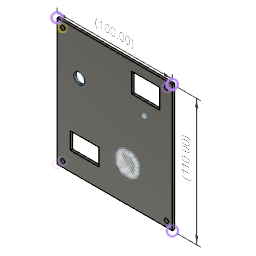
enclosure (Autodesk Fusion 360 archive; units mm, degrees)
design "Untitled"
part number: 2025-12-20-12-13-13-298
Autodesk Fusion 360 part; units mm, degrees
sketch "Sketch1" plane through (0, 0, 0) normal (0, 1, 0) x (1, 0, 0)
  line L0 (-50, -50) -> (40, -50)
  line L1 (40, -50) -> (40, 50)
  line L2 (40, 50) -> (-50, 50)
  line L3 (-50, 50) -> (-50, -50)
  dimension "d1" = 90
  dimension "d2" = 100
  constraint horizontal L0
  constraint vertical L1
  constraint horizontal L2
  constraint vertical L3
  measures "d1" distance of L0.start L0.end
  measures "d2" distance of L0.start L2.end
sketch "Sketch2" plane through (0, 0, 0) normal (0, 1, 0) x (1, 0, 0)
sketch "Sketch3" plane through (0, 0, 0) normal (0, 1, 0) x (1, 0, 0)
sketch "Sketch4" plane through (0, 0, 0) normal (0, 1, 0) x (1, 0, 0)
  line L0 (-43.399, 24.1645) -> (-18.699, 24.1645)
  line L1 (-18.699, 24.1645) -> (-18.699, 38.7645)
  line L2 (-18.699, 38.7645) -> (-43.399, 38.7645)
  line L3 (-43.399, 38.7645) -> (-43.399, 24.1645)
  dimension "d10" = 24.7
  dimension "d11" = 14.6
  constraint horizontal L0
  constraint vertical L1
  constraint horizontal L2
  constraint vertical L3
  measures "d10" distance of L0.start L0.end
  measures "d11" distance of L0.start L2.end
sketch "Sketch5" plane through (0, 0, 0) normal (0, 1, 0) x (1, 0, 0)
  circle A0 centre (-35.7, -19.12) radius 4.784
  circle A1 centre (0, 17) radius 0.35
  circle A2 centre (1, 18) radius 0.35
  circle A3 centre (2, 19) radius 0.35
  circle A4 centre (3, 20) radius 0.35
  circle A5 centre (4, 21) radius 0.35
  circle A6 centre (5, 22) radius 0.35
  circle A7 centre (6, 23) radius 0.35
  circle A8 centre (7, 24) radius 0.35
  circle A9 centre (8, 25) radius 0.35
  circle A10 centre (9, 26) radius 0.35
  circle A11 centre (10, 27) radius 0.35
  circle A12 centre (11, 28) radius 0.35
  circle A13 centre (12, 29) radius 0.35
  circle A14 centre (13, 30) radius 0.35
  circle A15 centre (1.9315, 15.9772) radius 0.35
  circle A16 centre (2.9315, 16.9772) radius 0.35
  circle A17 centre (3.9315, 17.9772) radius 0.35
  circle A18 centre (4.9315, 18.9772) radius 0.35
  circle A19 centre (5.9315, 19.9772) radius 0.35
  circle A20 centre (6.9315, 20.9772) radius 0.35
  circle A21 centre (7.9315, 21.9772) radius 0.35
  circle A22 centre (8.9315, 22.9772) radius 0.35
  circle A23 centre (1, 18) radius 0.35
  circle A24 centre (11.9315, 25.9772) radius 0.35
  circle A25 centre (10.9315, 24.9772) radius 0.35
  circle A26 centre (9.9315, 23.9772) radius 0.35
  circle A27 centre (12.9315, 26.9772) radius 0.35
  circle A28 centre (13.9315, 27.9772) radius 0.35
  circle A29 centre (13.9315, 24.9772) radius 0.35
  circle A30 centre (12.9315, 23.9772) radius 0.35
  circle A31 centre (11.9315, 22.9772) radius 0.35
  circle A32 centre (10.9315, 21.9772) radius 0.35
  circle A33 centre (9.9315, 20.9772) radius 0.35
  circle A34 centre (8.9315, 19.9772) radius 0.35
  circle A35 centre (7.9315, 18.9772) radius 0.35
  circle A36 centre (6.9315, 17.9772) radius 0.35
  circle A37 centre (5.9315, 16.9772) radius 0.35
  circle A38 centre (4.9315, 15.9772) radius 0.35
  circle A39 centre (3.9315, 14.9772) radius 0.35
  circle A40 centre (14.9315, 25.9772) radius 0.35
  circle A41 centre (6.9315, 14.9772) radius 0.35
  circle A42 centre (7.9315, 15.9772) radius 0.35
  circle A43 centre (8.9315, 16.9772) radius 0.35
  circle A44 centre (9.9315, 17.9772) radius 0.35
  circle A45 centre (10.9315, 18.9772) radius 0.35
  circle A46 centre (11.9315, 19.9772) radius 0.35
  circle A47 centre (12.9315, 20.9772) radius 0.35
  circle A48 centre (13.9315, 21.9772) radius 0.35
  circle A49 centre (14.9315, 22.9772) radius 0.35
  circle A50 centre (14.9315, 19.9772) radius 0.35
  circle A51 centre (13.9315, 18.9772) radius 0.35
  circle A52 centre (12.9315, 17.9772) radius 0.35
  circle A53 centre (11.9315, 16.9772) radius 0.35
  circle A54 centre (10.9315, 15.9772) radius 0.35
  circle A55 centre (9.9315, 14.9772) radius 0.35
  circle A56 centre (10.9315, 30.9772) radius 0.35
  circle A57 centre (9.9315, 29.9772) radius 0.35
  circle A58 centre (8.9315, 28.9772) radius 0.35
  circle A59 centre (7.9315, 27.9772) radius 0.35
  circle A60 centre (6.9315, 26.9772) radius 0.35
  circle A61 centre (5.9315, 25.9772) radius 0.35
  circle A62 centre (4.9315, 24.9772) radius 0.35
  circle A63 centre (3.9315, 23.9772) radius 0.35
  circle A64 centre (2.9315, 22.9772) radius 0.35
  circle A65 centre (1.9315, 21.9772) radius 0.35
  circle A66 centre (0.9315, 20.9772) radius 0.35
  circle A67 centre (-0.0685, 19.9772) radius 0.35
  circle A68 centre (-1.0685, 18.9772) radius 0.35
  circle A69 centre (-2.0685, 20.9772) radius 0.35
  circle A70 centre (-1.0685, 21.9772) radius 0.35
  circle A71 centre (-0.0685, 22.9772) radius 0.35
  circle A72 centre (0.9315, 23.9772) radius 0.35
  circle A73 centre (1.9315, 24.9772) radius 0.35
  circle A74 centre (2.9315, 25.9772) radius 0.35
  circle A75 centre (3.9315, 26.9772) radius 0.35
  circle A76 centre (4.9315, 27.9772) radius 0.35
  circle A77 centre (5.9315, 28.9772) radius 0.35
  circle A78 centre (6.9315, 29.9772) radius 0.35
  circle A79 centre (7.9315, 30.9772) radius 0.35
  circle A80 centre (8.9315, 31.9772) radius 0.35
  circle A81 centre (-2.0685, 23.9772) radius 0.35
  circle A82 centre (-1.0685, 24.9772) radius 0.35
  circle A83 centre (-0.0685, 25.9772) radius 0.35
  circle A84 centre (0.9315, 26.9772) radius 0.35
  circle A85 centre (1.9315, 27.9772) radius 0.35
  circle A86 centre (2.9315, 28.9772) radius 0.35
  circle A87 centre (3.9315, 29.9772) radius 0.35
  circle A88 centre (4.9315, 30.9772) radius 0.35
  circle A89 centre (5.9315, 31.9772) radius 0.35
  circle A90 centre (-2.0685, 26.9772) radius 0.35
  circle A91 centre (-1.0685, 27.9772) radius 0.35
  circle A92 centre (-0.0685, 28.9772) radius 0.35
  circle A93 centre (0.9315, 29.9772) radius 0.35
  circle A94 centre (1.9315, 30.9772) radius 0.35
  circle A95 centre (2.9315, 31.9772) radius 0.35
  dimension "d16" = 9.568
  dimension "d20" = 0.7
  dimension "d21" = 0.7
  dimension "d22" = 0.7
  dimension "d23" = 0.7
  dimension "d24" = 0.7
  dimension "d25" = 0.7
  dimension "d26" = 0.7
  dimension "d27" = 0.7
  dimension "d28" = 0.7
  dimension "d29" = 0.7
  dimension "d30" = 0.7
  dimension "d31" = 0.7
  dimension "d32" = 0.7
  dimension "d33" = 0.7
  dimension "d34" = 0.7
  dimension "d35" = 0.7
  dimension "d36" = 0.7
  dimension "d37" = 0.7
  dimension "d38" = 0.7
  dimension "d39" = 0.7
  dimension "d40" = 0.7
  dimension "d41" = 0.7
  dimension "d42" = 0.7
  dimension "d43" = 0.7
  dimension "d44" = 0.7
  dimension "d45" = 0.7
  dimension "d46" = 0.7
  dimension "d47" = 0.7
  dimension "d48" = 0.7
  dimension "d49" = 0.7
  dimension "d50" = 0.7
  dimension "d51" = 0.7
  dimension "d52" = 0.7
  dimension "d53" = 0.7
  dimension "d54" = 0.7
  dimension "d55" = 0.7
  dimension "d56" = 0.7
  dimension "d57" = 0.7
  dimension "d58" = 0.7
  dimension "d59" = 0.7
  dimension "d60" = 0.7
  dimension "d61" = 0.7
  dimension "d62" = 0.7
  dimension "d63" = 0.7
  dimension "d64" = 0.7
  dimension "d65" = 0.7
  dimension "d66" = 0.7
  dimension "d67" = 0.7
  dimension "d68" = 0.7
  dimension "d71" = 0.7
  dimension "d72" = 0.7
  dimension "d73" = 0.7
  dimension "d74" = 0.7
  dimension "d75" = 0.7
  dimension "d76" = 0.7
  dimension "d77" = 0.7
  dimension "d78" = 0.7
  dimension "d79" = 0.7
  dimension "d80" = 0.7
  dimension "d81" = 0.7
  dimension "d82" = 0.7
  dimension "d83" = 0.7
  dimension "d84" = 0.7
  dimension "d85" = 0.7
  dimension "d86" = 0.7
  dimension "d87" = 0.7
  dimension "d88" = 0.7
  dimension "d89" = 0.7
  dimension "d90" = 0.7
  dimension "d91" = 0.7
  dimension "d92" = 0.7
  dimension "d93" = 0.7
  dimension "d94" = 0.7
  dimension "d95" = 0.7
  dimension "d96" = 0.7
  dimension "d97" = 0.7
  dimension "d98" = 0.7
  dimension "d99" = 0.7
  dimension "d100" = 0.7
  dimension "d101" = 0.7
  dimension "d102" = 0.7
  dimension "d103" = 0.7
  dimension "d104" = 0.7
  dimension "d105" = 0.7
  dimension "d106" = 0.7
  dimension "d107" = 0.7
  dimension "d108" = 0.7
  dimension "d109" = 0.7
  dimension "d110" = 0.7
  dimension "d111" = 0.7
  dimension "d112" = 0.7
  dimension "d113" = 0.7
  dimension "d114" = 0.7
  dimension "d115" = 0.7
  dimension "d116" = 0.7
  measures "d16" diameter of A0
  measures "d20" diameter of A1
  measures "d21" diameter of A2
  measures "d22" diameter of A3
  measures "d23" diameter of A4
  measures "d24" diameter of A5
  measures "d25" diameter of A6
  measures "d26" diameter of A7
  measures "d27" diameter of A8
  measures "d28" diameter of A9
  measures "d29" diameter of A10
  measures "d30" diameter of A11
  measures "d31" diameter of A12
  measures "d32" diameter of A13
  measures "d33" diameter of A14
  measures "d34" diameter of A15
  measures "d35" diameter of A16
  measures "d36" diameter of A17
  measures "d37" diameter of A18
  measures "d38" diameter of A19
  measures "d39" diameter of A20
  measures "d40" diameter of A21
  measures "d41" diameter of A22
  measures "d42" diameter of A23
  measures "d43" diameter of A26
  measures "d44" diameter of A25
  measures "d45" diameter of A24
  measures "d46" diameter of A27
  measures "d47" diameter of A28
  measures "d48" diameter of A39
  measures "d49" diameter of A38
  measures "d50" diameter of A37
  measures "d51" diameter of A36
  measures "d52" diameter of A35
  measures "d53" diameter of A34
  measures "d54" diameter of A33
  measures "d55" diameter of A32
  measures "d56" diameter of A31
  measures "d57" diameter of A30
  measures "d58" diameter of A29
  measures "d59" diameter of A40
  measures "d60" diameter of A41
  measures "d61" diameter of A42
  measures "d62" diameter of A43
  measures "d63" diameter of A44
  measures "d64" diameter of A45
  measures "d65" diameter of A46
  measures "d66" diameter of A47
  measures "d67" diameter of A48
  measures "d68" diameter of A49
  measures "d71" diameter of A54
  measures "d72" diameter of A53
  measures "d73" diameter of A52
  measures "d74" diameter of A51
  measures "d75" diameter of A50
  measures "d76" diameter of A55
  measures "d77" diameter of A68
  measures "d78" diameter of A67
  measures "d79" diameter of A66
  measures "d80" diameter of A65
  measures "d81" diameter of A64
  measures "d82" diameter of A63
  measures "d83" diameter of A62
  measures "d84" diameter of A61
  measures "d85" diameter of A60
  measures "d86" diameter of A59
  measures "d87" diameter of A58
  measures "d88" diameter of A57
  measures "d89" diameter of A56
  measures "d90" diameter of A69
  measures "d91" diameter of A70
  measures "d92" diameter of A71
  measures "d93" diameter of A72
  measures "d94" diameter of A73
  measures "d95" diameter of A74
  measures "d96" diameter of A75
  measures "d97" diameter of A76
  measures "d98" diameter of A77
  measures "d99" diameter of A78
  measures "d100" diameter of A79
  measures "d101" diameter of A80
  measures "d102" diameter of A81
  measures "d103" diameter of A82
  measures "d104" diameter of A83
  measures "d105" diameter of A84
  measures "d106" diameter of A85
  measures "d107" diameter of A86
  measures "d108" diameter of A87
  measures "d109" diameter of A88
  measures "d110" diameter of A89
  measures "d111" diameter of A91
  measures "d112" diameter of A92
  measures "d113" diameter of A93
  measures "d114" diameter of A94
  measures "d115" diameter of A95
  measures "d116" diameter of A90
sketch "Sketch6" plane through (0, 0, 0) normal (0, 1, 0) x (1, 0, 0)
  circle A0 centre (20.89, -19.3) radius 0.8835
  dimension "d119" = 1.767
  measures "d119" diameter of A0
sketch "Sketch7" plane through (0, 0, 0) normal (0, 1, 0) x (1, 0, 0)
  line L0 (9.8, -47.2127) -> (34, -47.2127)
  line L1 (34, -47.2127) -> (34, -30.2127)
  line L2 (34, -30.2127) -> (9.8, -30.2127)
  line L3 (9.8, -30.2127) -> (9.8, -47.2127)
  constraint horizontal L0
  constraint vertical L1
  constraint horizontal L2
  constraint vertical L3
extrude "Extrude1" add sketch "Sketch1" along normal blind 2
sketch "Sketch8" plane through (0, 0, 0) normal (0, 1, 0) x (1, 0, 0)
  point P0 (-50, -50)
  point P1 (-50, 50)
  point P2 (40, -50)
  dimension "d131" = 100
  dimension "d132" = 90
  measures "d131" distance of P0 P1
  measures "d132" distance of P0 P2
sketch "Sketch9" plane through (0, 0, 0) normal (0, 1, 0) x (1, 0, 0)
sketch "Sketch10" plane through (0, 0, 0) normal (0, 1, 0) x (1, 0, 0)
sketch "Sketch11" plane through (0, 0, 0) normal (0, 1, 0) x (1, 0, 0)
sketch "Sketch12" plane through (0, 0, 0) normal (0, 1, 0) x (1, 0, 0)
  line L0 (-55, -55) -> (45, -55)
  line L1 (45, -55) -> (45, 55)
  line L2 (45, 55) -> (-55, 55)
  line L3 (-55, 55) -> (-55, -55)
  constraint horizontal L0
  constraint vertical L1
  constraint horizontal L2
  constraint vertical L3
extrude "Extrude2" add sketch "Sketch12" along normal blind 2
sketch "Sketch13" plane through (0, 0, 0) normal (0, 1, 0) x (1, 0, 0)
  point P0 (-55, -55)
  point P1 (45, -55)
  point P2 (-55, 55)
  dimension "d152" = 100
  dimension "d153" = 110
  measures "d152" distance of P0 P1
  measures "d153" distance of P0 P2
sketch "Sketch14" plane through (0, 0, 0) normal (0, 1, 0) x (1, 0, 0)
  line L0 (-49.3432, -49.6395) -> (38.5182, -49.6395)
  line L1 (38.5182, -49.6395) -> (38.5182, 49.7036)
  line L2 (38.5182, 49.7036) -> (-49.3432, 49.7036)
  line L3 (-49.3432, 49.7036) -> (-49.3432, -49.6395)
  constraint horizontal L0
  constraint vertical L1
  constraint horizontal L2
  constraint vertical L3
extrude "Extrude3" add sketch "Sketch14" along normal blind 2
extrude "Extrude4" cut sketch "Sketch7" sketch "Sketch4" sketch "Sketch5" along normal blind 75 of sketch 2 of sketch 3 contours A0
extrude "Extrude5" cut sketch "Sketch5" along normal blind 15 contours A1 | A2 A23 | A3 | A4 | A5 | A6 | A7 | A8 | A9 | A10 | A11 | A12 | A13 | A14 | A15 | A16 | A17 | A18 | A19 | A20 | A21 | A22 | A24 | A25 | A26 | A27 | A28 | A29 | A30 | A31 | A32 | A33 | A34 | A35 | A36 | A37 | A38 | A39 | A40 | A41 | A42 | A43 | A44 | A45 | A46 | A47 | A48 | A49 | A50 | A51 | A52 | A53 | A54 | A55 | A56 | A57 | A58 | A59 | A60 | A61 | A62 | A63 | A64 | A65 | A66 | A67 | A68 | A69 | A70 | A71 | A72 | A73 | A74 | A75 | A76 | A77 | A78 | A79 | A80 | A81 | A82 | A83 | A84 | A85 | A86 | A87 | A88 | A89 | A90 | A91 | A92 | A93 | A94 | A95
sketch "Sketch15" plane through (0, 0, 0) normal (0, 1, 0) x (1, 0, 0)
sketch "Sketch16" plane through (0, 0, 0) normal (0, 1, 0) x (1, 0, 0)
  circle A0 centre (-50, -50) radius 1.75
  circle A1 centre (40, -50) radius 1.75
  circle A2 centre (-50, 50) radius 1.7
  circle A3 centre (40, 50) radius 1.75
  dimension "d170" = 3.5
  dimension "d172" = 3.5
  dimension "d173" = 3.4
  dimension "d174" = 3.5
  measures "d170" diameter of A0
  measures "d172" diameter of A1
  measures "d173" diameter of A2
  measures "d174" diameter of A3
extrude "Extrude6" cut sketch "Sketch16" along normal blind 8
sketch "Sketch17" plane through (0, 0, 0) normal (0, 1, 0) x (1, 0, 0)
  point P0 (-55, -55)
  point P1 (45, -55)
  point P2 (45, 55)
  dimension "d177" = 100
  dimension "d178" = 110
  measures "d177" distance of P0 P1
  measures "d178" distance of P1 P2
